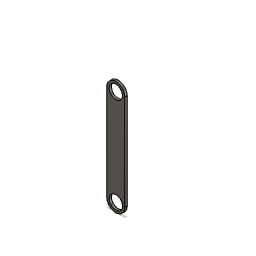
Joint 1 (Autodesk Fusion 360 design; units mm, degrees)
Autodesk Fusion 360 part; units mm, degrees
ref_plane "WorkPlane1" through (370, -25, 0) normal (0, 0, 1) x (1, 0, 0)
sketch "Sketch1" plane through (0, 0, 0) normal (0, 0, 1) x (1, 0, 0)
  circle A0 centre (356, -26.4187) radius 8.5
  line L0 (344.5, -26.4187) -> (344.5, -147.7874)
  line L1 (367.5, -26.4187) -> (367.5, -147.7874)
  arc A1 (367.5, -26.4187) -> (344.5, -26.4187) centre (356, -26.4187) ccw
  circle A2 centre (356, -147.7874) radius 8.5
  arc A3 (344.5, -147.7874) -> (367.5, -147.7874) centre (356, -147.7874) ccw
  point P0 (356, -147.7874)
  dimension "d103" = 17
  dimension "d104" = 23
  dimension "d105" = 17
  constraint concentric A0 A1
  constraint vertical L0
  constraint vertical L1
  constraint tangent L1 A1
  constraint tangent L0 A1
  constraint coincident P0 A2.centre
  constraint tangent L1 A3
  constraint concentric A2 A3
  measures "d103" diameter of A0
  measures "d104" diameter of A1
  measures "d105" diameter of A2
extrude "Extrude1" add sketch "Sketch1" along normal mid plane 40 contours A0
extrude "Extrude2" add sketch "Sketch1" along normal mid plane 3
extrude "Extrude3" cut 1 faces at (351.4712, -24.3078, 20) along direction (0, 0, -1) blind 54
